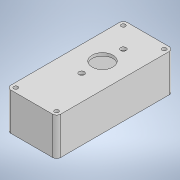
# Autodesk Inventor part: Голова сервы
Saved by Autodesk Inventor 2020 (Build 240168000, 168)
## iProperties
Created: 2021-09-05
Part Number: Голова сервы
Material: Типовые
Document SubType Name: Modeling
Designer: Антон
Density: 1 g/cm^3
Appearance: По умолчанию
Author: Антон
Autodesk Inventor part; units mm, degrees
ref_plane "YZ Plane" through (0, 0, 0) normal (1, 0, 0) x (0, 1, 0)
ref_plane "XZ Plane" through (0, 0, 0) normal (0, 1, 0) x (-1, 0, 0)
ref_plane "XY Plane" through (0, 0, 0) normal (0, 0, 1) x (1, 0, 0)
sketch "Эскиз1" plane through (0, 0, 0) normal (0, 1, 0) x (-1, 0, 0)
  line L0 (0, 0) -> (12, 0)
  line L1 (12, 0) -> (12, -28)
  line L2 (12, -28) -> (0, -28)
  line L3 (0, -28) -> (0, 0)
  circle A0 centre (6, -12) radius 0.65
  circle A1 centre (6, -17) radius 2.5
  circle A2 centre (6, -22) radius 0.65
  line L4 (6, -12) -> (6, -17) construction
  line L5 (6, -17) -> (6, -22) construction
  line L6 (6, -6) -> (6, 0) construction
  line L7 (6, -12) -> (12, -12) construction
  circle A3 centre (6, -12) radius 1.15
  circle A4 centre (6, -22) radius 1.15
  line L8 (6, -22) -> (6, -28) construction
  line L9 (6, -12) -> (6, -6) construction
  point P0 (12, -14)
  dimension "d0" = 5
  dimension "d1" = 6
  dimension "d2" = 5
  dimension "d7" = 0.5
  dimension "d8" = 1.3
  dimension "d20" = 6
  constraints: 20 end point, 5 centre point, 3 coincident, 3 equal length, 3 midpoint, 2 collinear, 2 equal radius, 2 parallel, 2 perpendicular, 2 point on line, 2 vertical, 1 concentric, 1 horizontal, 1 vertical alignment
  measures "d0" distance of L4.start L4.end
  measures "d1" distance of L4.start L7.end
  measures "d2" diameter of A1
  measures "d7" radial gap between concentric circles of A4 A2
  measures "d8" diameter of A2
  measures "d20" distance of L9.start L9.end
extrude "Выдавливание1" add sketch "Эскиз1" against normal blind 9 contours L0 L1 L2 L3 | A0 | A1 | A2 | A3 | A4
shell "Оболочка1" thickness 0.7 removed faces 1 at (-4, -9, -9.3333)
extrude "Выдавливание2" cut sketch "Эскиз1" against normal through all contours A0 | A1 | A2
sketch "Эскиз2" plane through (0, -9, 0) normal (0, -1, 0) x (1, 0, 0)
  line L0 (0, -28) -> (-12, -28) construction
  line L1 (-6, -28) -> (-6, 0) construction
  line L2 (-12, 0) -> (0, 0) construction
  line L3 (-12, -28) -> (-12, 0) construction
  line L4 (-12, -14) -> (0, -14) construction
  line L5 (0, 0) -> (0, -28) construction
  circle A0 centre (-1.1, -26.9) radius 0.9
  circle A1 centre (-1.1, -26.9) radius 0.5
  circle A2 centre (-10.9, -26.9) radius 0.9
  circle A3 centre (-10.9, -26.9) radius 0.5
  circle A4 centre (-1.1, -1.1) radius 0.9
  circle A5 centre (-1.1, -1.1) radius 0.5
  circle A6 centre (-10.9, -1.1) radius 0.5
  circle A7 centre (-10.9, -1.1) radius 0.9
  dimension "d11" = 1.1
  dimension "d12" = 1.1
  dimension "d13" = 1
  dimension "d14" = 0.4
  constraints: 8 centre point, 6 symmetric about line, 4 coincident, 4 end point, 4 midpoint, 6 other
  measures "d11" distance from line of L0 A0.centre
  measures "d12" distance from line of L5 A0.centre
  measures "d13" diameter of A1
  measures "d14" radial gap between concentric circles of A1 A0
extrude "Выдавливание3" cut sketch "Эскиз2" against normal through all contours A0 | A1 | A2 | A3 | A4 | A5 | A6 | A7
extrude "Выдавливание4" add sketch "Эскиз2" along normal blind 8.8 from surface at -9
fillet "Сопряжение1" radius 1 4 edges at (-12, -4.5, -28) (0, -4.5, -28) (0, -4.5, 0) (-12, -4.5, 0)
equation "\"d11\" = d12"
